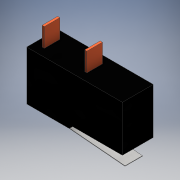
# Autodesk Inventor part: SS-5GL-F
Saved by Autodesk Inventor 2016 (Build 200138000, 138)
## iProperties
Created: 2016-01-29
Part Number: SS-5GL-F
Material: Generic
Document SubType Name: Modeling
Designer: jferner
Density: 1 g/cm^3
Appearance: Default
width: 6.400 mm
ss5glfLength: 19.800 mm
Author: jferner
Autodesk Inventor part; units mm, degrees
ref_plane "YZ Plane" through (0, 0, 0) normal (1, 0, 0) x (0, 1, 0)
ref_plane "XZ Plane" through (0, 0, 0) normal (0, 1, 0) x (-1, 0, 0)
sketch "Sketch1" plane through (0, 0, 0) normal (0, 1, 0) x (-1, 0, 0)
  line L0 (0, 0) -> (0, -10.2)
  line L1 (0, -10.2) -> (-8.8, -10.2)
  line L2 (-8.8, -10.2) -> (-9.5, -9.5)
  line L3 (-9.5, -9.5) -> (-19.8, -9.5)
  line L4 (-19.8, -9.5) -> (-19.8, 0)
  line L5 (-19.8, 0) -> (0, 0)
  dimension "d0" = 10.2
  dimension "d1" = 9.5
  dimension "ss5glfLength" = 19.8
  dimension "d4" = 8.8
  dimension "d5" = 135
  constraints: 12 end point, 3 perpendicular, 1 coincident, 1 parallel, 1 vertical
  measures "d0" distance of L0.start L0.end
  measures "d1" distance of L3.end L4.end
  measures "ss5glfLength" distance of L4.end L0.start
  measures "d4" distance of L0.end L1.end
  measures "d5" angle of L1 L2
extrude "Extrusion1" add sketch "Sketch1" along normal blind 6.4
sketch "Sketch2" plane through (0, 0, 0) normal (0, 0, 1) x (1, 0, 0)
  line L0 (1.6, 4.8) -> (2.06, 4.8)
  line L1 (2.06, 4.8) -> (2.06, 1.6)
  line L2 (2.06, 1.6) -> (1.6, 1.6)
  line L3 (1.6, 1.6) -> (1.6, 4.8)
  line L4 (10.4, 4.8) -> (10.86, 4.8)
  line L5 (10.86, 4.8) -> (10.86, 1.6)
  line L6 (10.86, 1.6) -> (10.4, 1.6)
  line L7 (10.4, 1.6) -> (10.4, 4.8)
  line L8 (0, 0) -> (0, 6.4) projected
  line L9 (19.8, 0) -> (0, 0) projected
  dimension "d8" = 0.46
  dimension "pinWidth" = 3.2
  dimension "d10" = 1.6
  dimension "d11" = 8.8
  dimension "d12" = 1.6
  constraints: 16 end point, 4 parallel, 2 horizontal, 2 perpendicular, 2 point on line, 1 collinear
  measures "d8" distance of L5.end L6.end
  measures "pinWidth" distance of L2.end L0.start
  measures "d10" distance between parallel lines of L8 L3
  measures "d11" distance between parallel lines of L7 L3
  measures "d12" distance between parallel lines of L9 L2
extrude "Extrusion2" add sketch "Sketch2" along normal blind 3.9
ref_plane "Work Plane1" through (0, 3.2, 0) normal (0, 1, 0) x (1, 0, 0)
sketch "Sketch3" plane through (0, 3.2, 0) normal (0, 1, 0) x (1, 0, 0)
  line L0 (8.8, 10.2) -> (0, 10.2) projected
  line L1 (3.1, 10.2) -> (3.1, 11.1084)
  line L2 (3.1, 11.1084) -> (18.9478, 12.4949)
  line L3 (18.9478, 12.4949) -> (18.9391, 12.5945)
  line L4 (18.9391, 12.5945) -> (3, 11.2)
  line L5 (3, 11.2) -> (3, 10.2)
  line L6 (0, 10.2) -> (0, 0) projected
  dimension "d15" = 16
  dimension "d16" = 1
  dimension "d17" = 0.1
  dimension "d18" = 0.1
  dimension "d19" = 95
  dimension "d20" = 3
  constraints: 10 end point, 2 perpendicular, 2 point on line, 1 parallel, 1 vertical
  measures "d15" distance of L3.end L4.end
  measures "d16" distance of L4.end L5.end
  measures "d17" distance of L2.end L3.end
  measures "d18" distance between parallel lines of L5 L1
  measures "d19" angle of L1 L2
  measures "d20" distance between parallel lines of L6 L5
extrude "Extrusion3" add sketch "Sketch3" along normal mid plane 3.6
equation "\"d12\" = -0.5 * pinWidth + 0.5 * width"
equation "\"width\" = 6.4"
body "Solid1"
